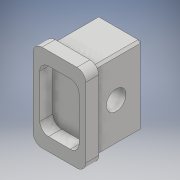
# Autodesk Inventor part: Steam Chest Slide Valve
Saved by Autodesk Inventor 2017 (Build 210142000, 142)
## iProperties
Created: 2018-11-17
Part Number: Steam Chest Slide Valve
Material: Generic
Document SubType Name: Modeling
Designer: Arman Grewal
Density: 1 g/cm^3
Appearance: Default
Author: Arman Grewal
Autodesk Inventor part; units mm, degrees
ref_plane "YZ Plane" through (0, 0, 0) normal (1, 0, 0) x (0, 1, 0)
ref_plane "XZ Plane" through (0, 0, 0) normal (0, 1, 0) x (-1, 0, 0)
ref_plane "XY Plane" through (0, 0, 0) normal (0, 0, 1) x (1, 0, 0)
sketch "Sketch1" plane through (0, 0, 0) normal (0, 1, 0) x (-1, 0, 0)
  line L0 (0, 0) -> (12, 0)
  line L1 (12, 0) -> (12, -20)
  line L2 (12, -20) -> (0, -20)
  line L3 (0, -20) -> (0, 0)
  dimension "d0" = 12
  dimension "d1" = 20
  constraints: 8 end point, 2 parallel, 1 horizontal, 1 perpendicular
  measures "d0" distance of L1.end L2.end
  measures "d1" distance of L0.end L1.end
extrude "Extrusion1" add sketch "Sketch1" along normal blind 3
sketch "Sketch2" plane through (0, 3, 0) normal (0, 1, 0) x (1, 0, 0)
  line L0 (-12, 20) -> (-12, 0) construction
  line L1 (-12, 10) -> (0, 10) construction
  line L2 (0, 0) -> (0, 20) construction
  line L3 (-1, 1) -> (-11, 1) construction
  line L4 (-11, 1) -> (-11, 19) construction
  line L5 (-11, 19) -> (-1, 19) construction
  line L6 (-1, 19) -> (-1, 1) construction
  line L7 (-1, 1) -> (-11, 19) construction
  line L8 (-11, 1) -> (-1, 19) construction
  line L9 (-1, 1) -> (-11, 1)
  line L10 (-11, 1) -> (-11, 19)
  line L11 (-11, 19) -> (-1, 19)
  line L12 (-1, 19) -> (-1, 1)
  line L13 (-1, 1) -> (-11, 19) construction
  line L14 (-11, 1) -> (-1, 19) construction
  point P0 (-6, 10)
  point P1 (-6, 10)
  dimension "d4" = 10
  dimension "d5" = 18
  constraints: 26 end point, 8 midpoint, 4 parallel, 2 horizontal, 2 perpendicular
  measures "d4" distance of L4.end L5.end
  measures "d5" distance of L3.end L4.end
extrude "Extrusion2" add sketch "Sketch2" along normal blind 11
sketch "Sketch3" plane through (-1, 3, -1) normal (1, 0, 0) x (0, 0, -1)
  line L0 (19, -3) -> (-1, -3) construction
  line L1 (9, -3) -> (9, 5) construction
  circle A0 centre (9, 5) radius 2.25
  dimension "d8" = 8
  dimension "d9" = 4.5
  constraints: 2 end point, 1 centre point, 1 coincident, 1 midpoint, 1 vertical
  measures "d8" distance of L1.start L1.end
  measures "d9" diameter of A0
extrude "Extrusion3" cut sketch "Sketch3" against normal blind 10
sketch "Sketch4" plane through (0, 0, 0) normal (0, -1, 0) x (1, 0, 0)
  line L0 (0, 0) -> (0, -20) construction
  line L1 (0, -10) -> (-12, -10) construction
  line L2 (-12, -20) -> (-12, 0) construction
  line L3 (-10.5, -3) -> (-1.5, -3) construction
  line L4 (-1.5, -3) -> (-1.5, -17) construction
  line L5 (-1.5, -17) -> (-10.5, -17) construction
  line L6 (-10.5, -17) -> (-10.5, -3) construction
  line L7 (-10.5, -3) -> (-1.5, -17) construction
  line L8 (-1.5, -3) -> (-10.5, -17) construction
  line L9 (-1.5, -3) -> (-10.5, -3) construction
  line L10 (-10.5, -3) -> (-10.5, -17) construction
  line L11 (-10.5, -17) -> (-1.5, -17) construction
  line L12 (-1.5, -17) -> (-1.5, -3) construction
  line L13 (-1.5, -3) -> (-10.5, -3)
  line L14 (-10.5, -3) -> (-10.5, -17)
  line L15 (-10.5, -17) -> (-1.5, -17)
  line L16 (-1.5, -17) -> (-1.5, -3)
  point P0 (-6, -10)
  dimension "d12" = 9
  dimension "d13" = 14
  constraints: 30 end point, 6 parallel, 5 midpoint, 3 horizontal, 3 perpendicular
  measures "d12" distance of L4.end L5.end
  measures "d13" distance of L3.end L4.end
extrude "Extrusion4" cut sketch "Sketch4" against normal blind 3
fillet "Fillet1" radius 2 8 edges at (-1.5, 1.5, -3) (-1.5, 1.5, -17) (-10.5, 1.5, -3) (-10.5, 1.5, -17) (0, 1.5, 0) (0, 1.5, -20) (-12, 1.5, 0) (-12, 1.5, -20)
chamfer "Chamfer1" distance 0.5 angle 45 8 edges at (-1, 8.5, -1) (-11, 14, -10) (-1, 8.5, -19) (-11, 8.5, -19) (-11, 8.5, -1) (-6, 14, -1) (-6, 14, -19) (-1, 14, -10)
body "Solid1"
